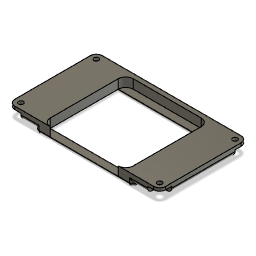
Top A v6 fix v2 (Autodesk Fusion 360 design; units mm, degrees)
Autodesk Fusion 360 part; units mm, degrees
sketch "スケッチ1" plane through (0, 0, 0) normal (0, 1, 0) x (1, 0, 0)
  line L0 (-100, 0) -> (100, 0) construction
  line L1 (0, 100) -> (0, -150) construction
  line L2 (-40, 40) -> (40, 40)
  line L3 (40, 40) -> (40, -40)
  line L4 (40, -40) -> (-40, -40)
  line L5 (-40, -40) -> (-40, 40)
  line L6 (-40, 7.5) -> (-12, 7.5)
  line L7 (-12, 7.5) -> (-12, -7.5)
  line L8 (-12, -7.5) -> (-40, -7.5)
  line L9 (-40, -7.5) -> (-40, 7.5)
  circle A0 centre (-35, 0) radius 2.5
  circle A1 centre (-20, 0) radius 2.5
  circle A2 centre (0, 0) radius 35 construction
  circle A3 centre (0, 0) radius 40 construction
  circle A4 centre (-35, 35) radius 1.25
  circle A5 centre (35, 35) radius 1.25
  circle A6 centre (-35, -35) radius 1.25
  circle A7 centre (35, -35) radius 1.25
  circle A8 centre (-35, 0) radius 5
  circle A9 centre (-20, 0) radius 5
  line L10 (-50, -52) -> (50, -52)
  line L11 (50, -52) -> (50, 50)
  line L12 (50, 50) -> (-50, 50)
  line L13 (-50, 50) -> (-50, -52)
  line L14 (50, -52) -> (-50, -52)
  line L15 (-50, -52) -> (-50, -110)
  line L16 (-50, -110) -> (50, -110)
  line L17 (50, -110) -> (50, -52)
  line L18 (27.5, -110) -> (-27.5, -110)
  line L19 (-27.5, -110) -> (-27.5, -55)
  line L20 (-27.5, -55) -> (27.5, -55)
  line L21 (27.5, -55) -> (27.5, -110)
  line L22 (48, -54) -> (48, -108)
  line L23 (48, -108) -> (-48, -108)
  line L24 (-48, -108) -> (-48, -54)
  line L25 (43, -43) -> (-43, -43)
  line L26 (-43, -43) -> (-43, 43)
  line L27 (-43, 43) -> (43, 43)
  line L28 (43, 43) -> (43, -43)
  line L29 (-40, -7.5) -> (-43, -7.5)
  line L30 (-40, 7.5) -> (-43, 7.5)
  line L31 (45, -45) -> (-45, -45)
  line L32 (-45, -45) -> (-45, 45)
  line L33 (-45, 45) -> (45, 45)
  line L34 (45, 45) -> (45, -45)
  line L35 (48, -54) -> (-48, -54)
  line L36 (10, -55) -> (10, -40)
  line L37 (-10, -55) -> (-10, -40)
  circle A10 centre (46, -106) radius 1.6
  circle A11 centre (46, -56) radius 1.6
  circle A12 centre (-46, -106) radius 1.6
  circle A13 centre (-46, -56) radius 1.6
  circle A14 centre (46, -106) radius 4
  circle A15 centre (46, -56) radius 4
  circle A16 centre (-46, -106) radius 4
  circle A17 centre (-46, -56) radius 4
  line L38 (36.7, -77) -> (-39.3, -77) construction
  line L39 (-39.3, -77) -> (-39.3, -61) construction
  line L40 (-39.3, -61) -> (36.7, -61) construction
  line L41 (36.7, -61) -> (36.7, -77) construction
  circle A18 centre (36.7, -61) radius 0.9
  circle A19 centre (36.7, -61) radius 4
  circle A20 centre (36.7, -77) radius 0.9
  circle A21 centre (36.7, -77) radius 4
  circle A22 centre (-39.3, -61) radius 0.9
  circle A23 centre (-39.3, -61) radius 4
  circle A24 centre (-39.3, -77) radius 0.9
  circle A25 centre (-39.3, -77) radius 4
  line L42 (27.5, -100) -> (-27.5, -100)
  line L43 (-42.127, -107) -> (42.127, -107)
  line L44 (-47, -102.127) -> (-47, -59.873)
  line L45 (47, -102.127) -> (47, -59.873)
  line L46 (-42.127, -55) -> (42.127, -55)
  arc A26 (-27.5, -105) -> (-22.5, -110) centre (-22.5, -105) ccw
  arc A27 (-22.5, -55) -> (-27.5, -60) centre (-22.5, -60) ccw
  arc A28 (27.5, -60) -> (22.5, -55) centre (22.5, -60) ccw
  arc A29 (22.5, -110) -> (27.5, -105) centre (22.5, -105) ccw
  line L47 (-35.3, -77) -> (-35.3, -61)
  line L48 (-43.3, -77) -> (-43.3, -61)
  line L49 (32.7, -77) -> (32.7, -61)
  line L50 (40.7, -77) -> (40.7, -61)
  line L51 (-46, -102) -> (-50, -102)
  line L52 (-42, -106) -> (-42, -110)
  line L53 (46, -102) -> (50, -102)
  line L54 (42, -106) -> (42, -110)
  line L55 (42, -56) -> (42, -52)
  line L56 (46, -60) -> (50, -60)
  line L57 (-42, -56) -> (-42, -52)
  line L58 (-46, -60) -> (-50, -60)
  line L59 (32.5, -110) -> (22.5, -110)
  line L60 (22.5, -110) -> (22.5, -55)
  line L61 (22.5, -55) -> (30, -55)
  line L62 (32.5, -57.5) -> (32.5, -110)
  line L63 (-30, -60) -> (32.5, -60)
  line L64 (32.5, -60) -> (32.5, -54.5)
  line L65 (30, -52) -> (-30, -52)
  line L66 (-32.5, -54.5) -> (-32.5, -57.5)
  line L67 (-30, -110) -> (30, -110)
  line L68 (32.5, -107.5) -> (32.5, -105)
  line L69 (32.5, -105) -> (-30, -105)
  line L70 (-32.5, -107.5) -> (-32.5, -107.5)
  arc A30 (-30, -105) -> (-32.5, -107.5) centre (-30, -107.5) ccw
  arc A31 (-32.5, -107.5) -> (-30, -110) centre (-30, -107.5) ccw
  arc A32 (30, -110) -> (32.5, -107.5) centre (30, -107.5) ccw
  arc A33 (-32.5, -57.5) -> (-30, -60) centre (-30, -57.5) ccw
  arc A34 (-30, -52) -> (-32.5, -54.5) centre (-30, -54.5) ccw
  arc A35 (32.5, -54.5) -> (30, -52) centre (30, -54.5) ccw
  dimension "d1" = 40
  dimension "d2" = 40
  dimension "d3" = 40
  dimension "d4" = 40
  dimension "d5" = 5
  dimension "d6" = 5
  dimension "d7" = 15
  dimension "d8" = 5
  dimension "d9" = 28
  dimension "d10" = 7.5
  dimension "d11" = 7.5
  dimension "d12" = 70
  dimension "d13" = 80
  dimension "d14" = 2.5
  dimension "d15" = 2.5
  dimension "d16" = 2.5
  dimension "d17" = 2.5
  dimension "d18" = 5
  dimension "d19" = 5
  dimension "d20" = 5
  dimension "d21" = 5
  dimension "d22" = 5
  dimension "d23" = 5
  dimension "d24" = 5
  dimension "d25" = 5
  dimension "d26" = 10
  dimension "d27" = 10
  dimension "d56" = 52
  dimension "d57" = 50
  dimension "d58" = 50
  dimension "d59" = 50
  dimension "d60" = 58
  dimension "d61" = 100
  dimension "d62" = 55
  dimension "d63" = 55
  dimension "d64" = 27.5
  dimension "d65" = 2
  dimension "d66" = 2
  dimension "d67" = 2
  dimension "d68" = 7
  dimension "d69" = 7
  dimension "d70" = 9
  dimension "d71" = 7
  dimension "d72" = 2
  dimension "d73" = 2
  dimension "d74" = 2
  dimension "d75" = 2
  dimension "d76" = 2
  dimension "d77" = 3.2
  dimension "d78" = 4
  dimension "d79" = 4
  dimension "d80" = 3.2
  dimension "d81" = 4
  dimension "d82" = 4
  dimension "d83" = 3.2
  dimension "d84" = 4
  dimension "d85" = 4
  dimension "d86" = 3.2
  dimension "d87" = 4
  dimension "d88" = 4
  dimension "d89" = 8
  dimension "d90" = 8
  dimension "d91" = 8
  dimension "d92" = 8
  dimension "d93" = 27.5
  dimension "d94" = 76
  dimension "d95" = 16
  dimension "d96" = 1.8
  dimension "d97" = 8
  dimension "d98" = 1.8
  dimension "d99" = 8
  dimension "d100" = 1.8
  dimension "d101" = 8
  dimension "d102" = 1.8
  dimension "d103" = 8
  dimension "d104" = 36.7
  dimension "d107" = 39.3
  dimension "d108" = 6
  dimension "d131" = 10
  dimension "d138" = 1
  dimension "d139" = 1
  dimension "d140" = 1
  dimension "d141" = 1
  dimension "d144" = 40
  dimension "d145" = 40
  dimension "d146" = 5
  dimension "d147" = 5
  dimension "d148" = 5
  dimension "d149" = 5
  dimension "d150" = 5
  dimension "d151" = 5
  dimension "d152" = 5
  dimension "d153" = 5
  dimension "d163" = 5
  dimension "d164" = 5
  dimension "d165" = 5
  dimension "d166" = 5
  dimension "d167" = 5
  dimension "d168" = 2.5
  dimension "d169" = 2.5
  dimension "d171" = 2.5
  dimension "d172" = 2.5
  dimension "d173" = 5
  dimension "d174" = 2.5
  constraint horizontal L0
  constraint perpendicular L0 L1
  constraint horizontal L2
  constraint vertical L3
  constraint horizontal L4
  constraint vertical L5
  constraint horizontal L6
  constraint vertical L7
  constraint horizontal L8
  constraint vertical L9
  constraint coincident L5 L6.start
  constraint coincident L0 A0.centre
  constraint coincident L0 A1.centre
  constraint coincident A2.centre A3.centre
  constraint concentric A2 A3
  constraint concentric A0 A8
  constraint concentric A1 A9
  constraint horizontal L10
  constraint vertical L11
  constraint horizontal L12
  constraint vertical L13
  constraint horizontal L14
  constraint vertical L15
  constraint horizontal L16
  constraint vertical L17
  constraint horizontal L18
  constraint vertical L19
  constraint horizontal L20
  constraint vertical L21
  constraint coincident L16 L18.start
  constraint perpendicular L16 L22
  constraint perpendicular L22 L23
  constraint perpendicular L10 L24
  constraint horizontal L25
  constraint vertical L26
  constraint horizontal L27
  constraint vertical L28
  constraint coincident L26 L29.end
  constraint perpendicular L26 L29
  constraint coincident L26 L30.end
  constraint perpendicular L26 L30
  constraint horizontal L31
  constraint vertical L32
  constraint horizontal L33
  constraint vertical L34
  constraint coincident L22 L35.start
  constraint coincident L24 L35.end
  constraint perpendicular L24 L35
  constraint coincident L4 L36.end
  constraint perpendicular L4 L36
  constraint coincident L4 L37.end
  constraint perpendicular L4 L37
  constraint concentric A10 A14
  constraint concentric A11 A15
  constraint concentric A12 A16
  constraint concentric A13 A17
  constraint horizontal L38
  constraint vertical L39
  constraint horizontal L40
  constraint vertical L41
  constraint coincident L40.end L41.start
  constraint concentric A18 A19
  constraint coincident L38.start L41.end
  constraint concentric A20 A21
  constraint coincident L39.end L40.start
  constraint concentric A22 A23
  constraint coincident L38.end L39.start
  constraint concentric A24 A25
  constraint perpendicular L19 L42
  constraint coincident L19 L42.end
  constraint coincident L21 L42.start
  constraint coincident A16 L43.start
  constraint coincident A14 L43.end
  constraint horizontal L43
  constraint coincident A16 L44.start
  constraint coincident A17 L44.end
  constraint vertical L44
  constraint coincident A14 L45.start
  constraint coincident A15 L45.end
  constraint parallel L22 L45
  constraint coincident A17 L46.start
  constraint coincident A15 L46.end
  constraint perpendicular L36 L46
  constraint coincident L37.start L46
  constraint coincident L36.start L46
  constraint coincident L18 A26.end
  constraint tangent L16 A26
  constraint coincident L20 A27.start
  constraint coincident L20 A28.end
  constraint coincident L18 A29.start
  constraint tangent L20 A27
  constraint tangent L20 A28
  constraint tangent L21 A29
  constraint coincident L38 L47.start
  constraint coincident A25 L47.start
  constraint coincident L40 L47.end
  constraint coincident A23 L47.end
  constraint coincident A25 L48.start
  constraint coincident A23 L48.end
  constraint tangent A23 L48
  constraint perpendicular L40 L48
  constraint coincident L38 L49.start
  constraint coincident A21 L49.start
  constraint coincident A19 L49.end
  constraint coincident L40 L49.end
  constraint coincident A21 L50.start
  constraint coincident A19 L50.end
  constraint tangent A19 L50
  constraint perpendicular L40 L50
  constraint coincident A16 L51.start
  constraint coincident L15 L51.end
  constraint perpendicular L15 L51
  constraint coincident A16 L52.start
  constraint coincident L16 L52.end
  constraint perpendicular L16 L52
  constraint tangent A16 L52
  constraint tangent A16 L51
  constraint coincident A14 L53.start
  constraint coincident L17 L53.end
  constraint perpendicular L17 L53
  constraint coincident A14 L54.start
  constraint coincident L16 L54.end
  constraint perpendicular L16 L54
  constraint coincident A15 L55.start
  constraint coincident L14 L55.end
  constraint perpendicular L14 L55
  constraint coincident A15 L56.start
  constraint coincident L17 L56.end
  constraint perpendicular L17 L56
  constraint coincident A17 L57.start
  constraint coincident L14 L57.end
  constraint tangent A17 L57
  constraint perpendicular L14 L57
  constraint coincident A17 L58.start
  constraint coincident L15 L58.end
  constraint perpendicular L15 L58
  constraint tangent A17 L58
  constraint tangent A15 L55
  constraint tangent A15 L56
  constraint tangent A14 L53
  constraint tangent A14 L54
  constraint horizontal L59
  constraint vertical L60
  constraint horizontal L61
  constraint vertical L62
  constraint coincident A28 L60.end
  constraint coincident L16 L59.start
  constraint horizontal L63
  constraint vertical L64
  constraint horizontal L65
  constraint vertical L66
  constraint horizontal L67
  constraint vertical L68
  constraint horizontal L69
  constraint coincident L62 L68.end
  constraint collinear L62 L64
  constraint tangent L69 A30
  constraint tangent L67 A31
  constraint equal A30 A31
  constraint collinear L16 L67
  constraint tangent L67 A32
  constraint tangent L68 A32
  constraint tangent L63 A33
  constraint tangent L66 A33
  constraint tangent L65 A34
  constraint tangent L66 A34
  constraint tangent L64 A35
  constraint tangent L65 A35
  measures "d1" distance of L0 L2
  measures "d2" distance of L0 L4
  measures "d3" distance of L1 L5
  measures "d4" distance of L1 L3
  measures "d5" diameter of A0
  measures "d6" diameter of A1
  measures "d7" distance of A0.centre A1.centre
  measures "d8" distance of L5 A0.centre
  measures "d9" distance of L7 L9
  measures "d10" distance of L0 L6
  measures "d11" distance of L0 L8
  measures "d12" diameter of A2
  measures "d13" diameter of A3
  measures "d14" diameter of A4
  measures "d15" diameter of A5
  measures "d16" diameter of A6
  measures "d17" diameter of A7
  measures "d18" distance of L2 A4.centre
  measures "d19" distance of L5 A4.centre
  measures "d20" distance of L2 A5.centre
  measures "d21" distance of L3 A5.centre
  measures "d22" distance of L4 A6.centre
  measures "d23" distance of L5 A6.centre
  measures "d24" distance of L3 A7.centre
  measures "d25" distance of L4 A7.centre
  measures "d26" diameter of A8
  measures "d27" diameter of A9
  measures "d56" distance of L0 L10
  measures "d57" distance of L0 L12
  measures "d58" distance of L1 L13
  measures "d59" distance of L1 L11
  measures "d60" distance of L14 L16
  measures "d61" distance of L15 L17
  measures "d62" distance of L19 L21
  measures "d63" distance of L18 L20
  measures "d64" distance of L1 L21
  measures "d65" distance of L17 L22
  measures "d66" distance of L16 L23
  measures "d67" distance of L15 L24
  measures "d68" distance of L11 L28
  measures "d69" distance of L12 L27
  measures "d70" distance of L14 L25
  measures "d71" distance of L13 L26
  measures "d72" distance of L27 L33
  measures "d73" distance of L28 L34
  measures "d74" distance of L25 L31
  measures "d75" distance of L26 L32
  measures "d76" distance of L10 L35
  measures "d77" diameter of A10
  measures "d78" distance of L16 A10.centre
  measures "d79" distance of L17 A10.centre
  measures "d80" diameter of A11
  measures "d81" distance of L17 A11.centre
  measures "d82" distance of L14 A11.centre
  measures "d83" diameter of A12
  measures "d84" distance of L15 A12.centre
  measures "d85" distance of L16 A12.centre
  measures "d86" diameter of A13
  measures "d87" distance of L15 A13.centre
  measures "d88" distance of L10 A13.centre
  measures "d89" diameter of A14
  measures "d90" diameter of A15
  measures "d91" diameter of A16
  measures "d92" diameter of A17
  measures "d93" distance of L1 L19
  measures "d94" distance of L39 L41
  measures "d95" distance of L38 L40
  measures "d96" diameter of A18
  measures "d97" diameter of A19
  measures "d98" diameter of A20
  measures "d99" diameter of A21
  measures "d100" diameter of A22
  measures "d101" diameter of A23
  measures "d102" diameter of A24
  measures "d103" diameter of A25
  measures "d104" distance of L1 L41
  measures "d107" distance of L1 L39
  measures "d108" distance of L20 L40
  measures "d131" distance of L16 L42
  measures "d138" distance of L22 L45
  measures "d139" distance of L23 L43
  measures "d140" distance of L24 L44
  measures "d141" distance of L35 L46
  measures "d144" distance of L11 L36
  measures "d145" distance of L13 L37
  measures "d146" distance of L16 A26.centre
  measures "d147" distance of L19 A26.centre
  measures "d148" distance of L16 A29.centre
  measures "d149" distance of L21 A29.centre
  measures "d150" distance of L20 A28.centre
  measures "d151" distance of L21 A28.centre
  measures "d152" distance of L20 A27.centre
  measures "d153" distance of L19 A27.centre
  measures "d163" distance of L67 L69
  measures "d164" distance of L21 L60
  measures "d165" distance of L21 L62
  measures "d166" distance of L46 L63
  measures "d167" distance of L19 L66
  measures "d168" radius of A30
  measures "d169" radius of A32
  measures "d171" radius of A33
  measures "d172" radius of A34
  measures "d173" distance of L19 L70.start
  measures "d174" radius of A35
extrude "押し出し16" add sketch "スケッチ1" along normal blind 6 contours L10 L14 L35 L36 L37 L65 | L10 L14 L35 L36 L65 A35 | L10 L14 L35 L37 L65 A34 | L10 L14 L35 L55 A35 | L10 L14 L35 L57 A34 | L10 L14 L35 A15 L55 | L10 L14 L35 A17 L57 | L22 L35 A15 | L24 L35 A17 | L17 L22 A15 L56 | L22 L35 A15 | L24 L35 A17 | L15 L24 A17 L58 | L17 L22 L53 L56 | L15 L24 L51 L58 | L17 L22 A14 L53 | L15 L24 A16 L51 | L22 L23 A14 | L23 L24 A16 | L22 L23 A14 | L16 L23 A14 L54 | L16 L21 L23 L59 L67 A32 | L16 L18 L21 L23 A29 L59 L67 | L23 L24 A16 | L16 L23 A16 L52 | L16 L18 L19 L23 A26 L67 | L16 L19 L23 L67 A31 | L16 L23 L54 L62 | L16 L23 L59 L62 A32 | L16 L23 L52 A31
extrude "押し出し17" add sketch "スケッチ1" along normal blind 6 contours L20 L35 L36 L37 L46 | L20 L35 L36 L46 L61 L64 A35 | L20 L35 L37 L46 L66 A34 | L35 L46 L55 L64 A35 | L35 L46 L57 L66 A34 | L35 A15 L46 L55 | L20 L21 L46 A28 L61 | L35 A17 L46 L57 | L19 L20 L46 A27 | A14 A15 L43 L45 L46 L53 L54 L55 L56 L62 L64 L68 | A15 L46 L55 | L21 L46 L61 L62 L63 L64 | L21 L62 L63 L69 | A17 L46 L57 | L19 A16 A17 L43 L44 L46 L51 L52 L57 L58 L63 L66 L69 A30 A33 | L19 L46 L63 L66 A33 | L22 A15 L45 L56 | L24 A17 L44 L58 | L22 L45 L53 L56 | A15 L45 L56 | L21 L43 L62 L68 L69 | L21 L43 A29 | L24 L44 L51 L58 | A17 L44 L58 | L19 L43 A26 | L19 L43 L69 A30 | L22 A14 L45 L53 | L21 L23 L43 L62 L68 A32 | L21 L23 L43 A29 | L23 L43 L54 L62 L68 | L24 A16 L44 L51 | L19 L23 L43 A26 | L19 L23 L43 A30 A31 | A14 L45 L53 | A14 L43 L54 | L23 A14 L43 L54 | L23 L62 A32 | A16 L44 L51 | L23 L43 L52 A30 A31 | L23 A16 L43 L52 | A16 L43 L52 | A18 | A19 | A19 A21 L49 L50 | A21 | A20 | A22 | A23 | A23 A25 L47 L48 | A25 | A24
extrude "押し出し18" cut sketch "スケッチ1" along normal blind 4 contours L10 L14 L35 A15 L55 | L10 L14 L35 A17 L57 | L22 L35 A15 | L35 A15 L46 L55 | L10 L14 L15 A17 | L24 L35 A17 | L35 A17 L46 L57 | L17 L22 A15 L56 | L22 L35 A15 | A15 L46 L55 | L24 L35 A17 | L15 L24 A17 L58 | A17 L46 L57 | L22 A15 L45 L56 | L24 A17 L44 L58 | L17 L22 A14 L53 | A15 L45 L56 | L15 L24 A16 L51 | A17 L44 L58 | L22 L23 A14 | L22 A14 L45 L53 | L23 L24 A16 | L24 A16 L44 L51 | L22 L23 A14 | L16 L23 A14 L54 | A14 L45 L53 | A14 L43 L54 | L23 A14 L43 L54 | L23 L24 A16 | L16 L23 A16 L52 | A16 L44 L51 | L23 A16 L43 L52 | A16 L43 L52
extrude "押し出し19" add sketch "スケッチ1" against normal blind 2 contours L10 L14 L35 L36 L37 L65 | L10 L14 L35 L36 L65 A35 | L10 L14 L35 L37 L65 A34 | L20 L35 L36 L37 L46 | L20 L35 L36 L46 L61 L64 A35 | L20 L35 L37 L46 L66 A34 | L20 L46 A27 L60 L63 | L20 L21 L46 A28 L61 | A28 L60 L63 | L19 L20 L46 A27 | L21 L46 L61 L62 L63 L64 | L21 L62 L63 L69 | L21 L42 L60 L63 | L19 L46 L63 L66 A33 | L21 L42 L60 L69 | L21 L43 L62 L68 L69 | L21 L43 A29 | L43 A29 L60 L69 | L43 A26 L60 L69 | L19 L43 A26 | L19 L43 L69 A30 | L21 L23 L43 L62 L68 A32 | L21 L23 L43 A29 | L23 L43 A29 L60 | L23 L43 A26 L60 | L19 L23 L43 A26 | L19 L23 L43 A30 A31 | L16 L21 L23 L59 L67 A32 | L16 L18 L21 L23 A29 L59 L67 | L23 A29 L60 | L16 L18 L23 A26 L60 L67 | L16 L18 L19 L23 A26 L67 | L16 L19 L23 L67 A31
fillet "フィレット8" radius 3 6 edges at (50, 0, 81) (36, 0, 110) (36, 0, 52) (-36, 0, 110) (-50, 0, 81) (-36, 0, 52)
fillet "フィレット9" radius 2 12 edges at (-3.75, -2, 60) (-31.7678, -2, 59.2678) (-32.5, -2, 56) (-31.7678, -2, 52.7322) (0, -2, 52) (31.7678, -2, 52.7322) (32.5, -2, 81) (31.7678, -2, 109.2678) (0, -2, 110) (-32.5, -2, 107.5) (-3.75, -2, 105) (22.5, -2, 82.5)
fillet "フィレット7" [suppressed]
extrude "押し出し1" [suppressed]
extrude "押し出し2" [suppressed]
extrude "押し出し8" [suppressed]
extrude "押し出し11" [suppressed]
extrude "押し出し12" [suppressed]
extrude "押し出し3" [suppressed]
fillet "フィレット1" [suppressed]
extrude "押し出し9" [suppressed]
extrude "押し出し10" [suppressed]
fillet "フィレット2" [suppressed]
fillet "フィレット3" [suppressed]
fillet "フィレット4" [suppressed]
extrude "押し出し13" [suppressed]
extrude "押し出し14" [suppressed]
fillet "フィレット6" [suppressed]
extrude "押し出し15" [suppressed]
